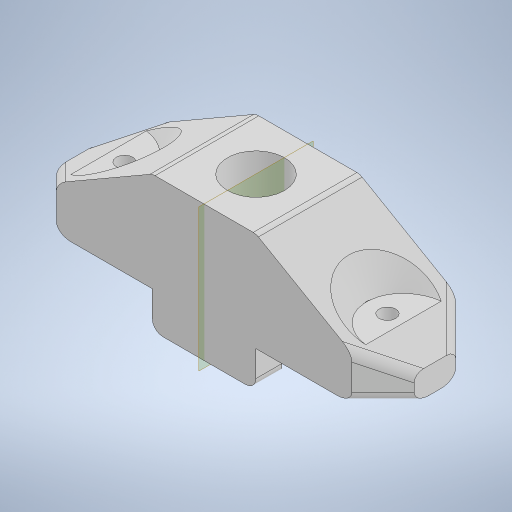
# Autodesk Inventor part: Belt tensioner mount
Saved by Autodesk Inventor 2023.1 (Build 271208000, 208)
## iProperties
Created: 2023-01-05
Part Number: Belt tensioner mount
Material: Generic
Document SubType Name: Modeling
Designer: nicol
Density: 1 g/cm^3
Appearance: Default
Author: nicol
Autodesk Inventor part; units mm, degrees
ref_plane "YZ Plane" through (0, 0, 0) normal (1, 0, 0) x (0, 1, 0)
ref_plane "XZ Plane" through (0, 0, 0) normal (0, 1, 0) x (-1, 0, 0)
sketch "Sketch1" plane through (0, 0, 0) normal (0, 0, 1) x (1, 0, 0)
  line L0 (0, 0) -> (0, 5)
  line L1 (0, 5) -> (24.5, 19.1451)
  line L2 (24.5, 19.1451) -> (44.5, 19.1451)
  line L3 (44.5, 19.1451) -> (69, 5)
  line L4 (69, 5) -> (69, 0)
  line L5 (69, 0) -> (44.5, 0)
  line L6 (44.5, 0) -> (44.5, -7)
  line L7 (44.5, -7) -> (24.5, -7)
  line L8 (24.5, -7) -> (24.5, 0)
  line L9 (24.5, 0) -> (0, 0)
  dimension "d0" = 20
  dimension "d1" = 7
  dimension "d2" = 5
  dimension "d3" = 24.5
  dimension "d4" = 120
  dimension "d5" = 120
  dimension "d6" = 20
  constraints: 20 end point, 4 parallel, 3 perpendicular, 2 equal length, 1 collinear, 1 vertical
  measures "d0" distance of L6.end L7.end
  measures "d1" distance of L7.end L8.end
  measures "d2" distance of L0.start L0.end
  measures "d3" distance of L8.end L0.start
  measures "d4" angle of L1 L0
  measures "d5" angle of L4 L3
  measures "d6" distance of L1.end L2.end
extrude "Extrusion1" add sketch "Sketch1" along normal blind 20
sketch "Sketch2" plane through (24.5, -7, 0) normal (0, -1, 0) x (1, 0, 0)
  line L0 (0, 0) -> (20, 0) projected
  line L1 (20, 0) -> (20, 20) projected
  line L2 (0, 20) -> (20, 20) projected
  line L3 (0, 0) -> (0, 20) projected
  line L4 (0, 15) -> (2.5, 12.5)
  line L5 (2.5, 12.5) -> (2.5, 7.5)
  line L6 (2.5, 7.5) -> (0, 5)
  point P0 (-24.5, 0)
  point P1 (0, 10)
  point P2 (2.5, 10)
  dimension "d9" = 135
  dimension "d10" = 135
  dimension "d11" = 10
  dimension "d12" = 2.5
  constraints: 6 end point, 2 midpoint, 2 point on line, 1 horizontal alignment, 1 vertical
  measures "d9" angle of L5 L4
  measures "d10" angle of L5 L6
  measures "d11" distance of L6.end L4.start
  measures "d12" distance between parallel lines of L3 L5
extrude "Extrusion2" cut sketch "Sketch2" against normal up to surface (7 mm away) contours L3 L4 L5 L6
ref_plane "Work Plane1" through (34.5, -7, 20) normal (-1, 0, 0) x (0, 0, 1)
sketch "Sketch3" plane through (0, 0, 0) normal (0, -1, 0) x (1, 0, 0)
  line L0 (24.5, 15) -> (24.5, 20) projected
  line L1 (0, 0) -> (0, 20) projected
  circle A0 centre (9.15, 10) radius 4
  circle A1 centre (9.15, 10) radius 1.6
  point P0 (0, 10)
  dimension "d15" = 15.35
  dimension "d16" = 3.2
  dimension "d17" = 8
  constraints: 2 centre point, 2 coincident, 1 horizontal alignment, 1 midpoint
  measures "d15" distance from line of L0 point (9.15, 10)
  measures "d16" diameter of A1
  measures "d17" diameter of A0
extrude "Extrusion3" cut sketch "Sketch3" against normal through all contours A1
ref_plane "Work Plane2" through (0, 8.5, 0) normal (0, -1, 0) x (1, 0, 0)
extrude "Extrusion4" cut sketch "Sketch3" against normal blind 10 from surface at -8.5
sketch "Sketch4" plane through (24.5, 19.1451, 0) normal (0, 1, 0) x (1, 0, 0)
  line L0 (20, 0) -> (0, 0) projected
  line L1 (0, 0) -> (0, -20) projected
  line L2 (20, -20) -> (0, -20) projected
  line L3 (20, 0) -> (20, -20) projected
  point P0 (-24.5, 0)
  point P1 (10, -10)
  point P2 (20, -10)
  point P3 (10, -20)
  constraints: 2 midpoint, 1 horizontal alignment, 1 vertical alignment
hole "Hole1" at (34.5, 19.1451, 10) direction (0, -1, 0) diameter 6.2 end through all counterbore diameter 11 counterbore depth 19
mirror "Mirror1" about plane through (34.5, -7, 20) normal (-1, 0, 0) of "Extrusion2", "Extrusion3", "Extrusion4"
chamfer "Chamfer1" distance 6 angle 45 4 edges at (0, 2.5, 0) (0, 2.5, 20) (69, 2.5, 20) (69, 2.5, 0)
fillet "Fillet1" radius 2 14 edges at (3, 0, 3) (24.5, -7, 2.5) (24.5, -7, 17.5) (3, 0, 17) (3, 6.7321, 17) (3, 6.7321, 3) (24.5, 19.1451, 10) (44.5, -7, 17.5) (44.5, -7, 2.5) (66, 6.7321, 17) (66, 0, 17) (66, 6.7321, 3) (66, 0, 3) (44.5, 19.1451, 10)
chamfer "Chamfer2" distance 4 angle 45 4 edges at (58.4993, 11.0626, 13.7651) (58.4993, 11.0626, 6.2349) (10.5007, 11.0626, 6.2349) (10.5007, 11.0626, 13.7651)
body "Solid1"
